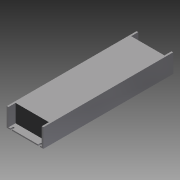
# Autodesk Inventor part: 5v_psu
Saved by Autodesk Inventor 2013 SP2 (Build 170200200, 200)
## iProperties
Created: 2018-10-22
Part Number: 5v_psu
Material: Generic
Document SubType Name: Modeling
Designer: alex
Density: 1 g/cm^3
Mass: 393.303 g
Surface Area: 466.03 cm^2
Volume: 393.303 cm^3
Author: alex
Autodesk Inventor part; units mm, degrees
ref_plane "YZ Plane" through (0, 0, 0) normal (1, 0, 0) x (0, 1, 0)
ref_plane "XZ Plane" through (0, 0, 0) normal (0, 1, 0) x (-1, 0, 0)
sketch "Sketch1" plane through (0, 0, 0) normal (0, 1, 0) x (-1, 0, 0)
  line L0 (34.1299, -113.6069) -> (-27.8701, -113.6069)
  line L1 (-27.8701, -113.6069) -> (-27.8701, 106.3931)
  line L2 (-27.8701, 106.3931) -> (34.1299, 106.3931)
  line L3 (34.1299, 106.3931) -> (34.1299, -113.6069)
  line L4 (34.1299, -113.6069) -> (-27.8701, 106.3931) construction
  line L5 (-27.8701, -113.6069) -> (34.1299, 106.3931) construction
  point P0 (0, 0)
  point P1 (3.1299, -3.6069)
  dimension "d0" = 62
  dimension "d1" = 220
  constraints: 12 end point, 2 midpoint, 2 parallel, 1 horizontal, 1 perpendicular
  measures "d0" distance of L1.end L2.end
  measures "d1" distance of L0.end L1.end
extrude "Extrusion1" add sketch "Sketch1" along normal blind 31.8
sketch "Sketch2" plane through (-34.1299, 0, 106.3931) normal (0, 0, 1) x (1, 0, 0)
  line L0 (62, 0) -> (0, 0) projected
  line L1 (62, 0) -> (62, 31.8) projected
  line L2 (0, 0) -> (0, 31.8) projected
  line L3 (2.8, 38.8076) -> (59.2, 38.8076)
  line L4 (59.2, 38.8076) -> (59.2, 2)
  line L5 (59.2, 2) -> (2.8, 2)
  line L6 (2.8, 2) -> (2.8, 38.8076)
  point P0 (34.1299, 0)
  dimension "d4" = 2.8
  dimension "d5" = 2.8
  dimension "d6" = 2
  constraints: 8 end point, 2 parallel, 1 horizontal, 1 perpendicular
  measures "d4" distance between parallel lines of L1 L4
  measures "d5" distance between parallel lines of L2 L6
  measures "d6" distance between parallel lines of L0 L5
extrude "Extrusion2" cut sketch "Sketch2" against normal blind 12
ref_plane "Work Plane1" through (27.8701, 0, -3.6069) normal (0, 0, -1) x (-1, 0, 0)
mirror "Mirror1" about plane through (27.8701, 0, -3.6069) normal (0, 0, -1) of "Extrusion2"
sketch "Sketch3" plane through (0, 0, 0) normal (0, -1, 0) x (1, 0, 0)
  line L0 (-34.1299, -113.6069) -> (27.8701, -113.6069) projected
  line L1 (27.8701, -113.6069) -> (27.8701, 106.3931) projected
  line L2 (27.8701, 106.3931) -> (-34.1299, 106.3931) projected
  line L3 (-34.1299, 106.3931) -> (-34.1299, -113.6069) projected
  line L4 (-26.6299, 106.3931) -> (-26.6299, 102.8931)
  circle A0 centre (-26.6299, 102.8931) radius 1.5
  line L5 (-28.1299, 102.8931) -> (-28.1299, 106.3931)
  line L6 (-25.1299, 102.8931) -> (-25.1299, 106.3931)
  line L7 (20.3701, 106.3931) -> (20.3701, 102.8931)
  circle A1 centre (20.3701, 102.8931) radius 1.5
  line L8 (21.8701, 102.8931) -> (21.8701, 106.3931)
  line L9 (18.8701, 102.8931) -> (18.8701, 106.3931)
  line L10 (-26.6299, -113.6069) -> (-26.6299, -110.1069)
  circle A2 centre (-26.6299, -110.1069) radius 1.5
  line L11 (-25.1299, -110.1069) -> (-25.1299, -113.6069)
  line L12 (-28.1299, -110.1069) -> (-28.1299, -113.6069)
  line L13 (20.3701, -113.6069) -> (20.3701, -110.1069)
  circle A3 centre (20.3701, -110.1069) radius 1.5
  line L14 (18.8701, -110.1069) -> (18.8701, -113.6069)
  line L15 (21.8701, -110.1069) -> (21.8701, -113.6069)
  point P0 (0, 0)
  dimension "d9" = 3
  dimension "d10" = 3.5
  dimension "d11" = 6
  dimension "d12" = 3.5
  dimension "d14" = 3
  dimension "d15" = 3.5
  dimension "d16" = 3
  dimension "d18" = 3.5
  dimension "d19" = 3
  dimension "d23" = 6
  dimension "d24" = 6
  dimension "d25" = 6
  constraints: 24 end point, 12 point on line, 9 perpendicular, 8 point on circle, 8 tangent, 4 centre point, 4 coincident, 3 parallel
  measures "d9" diameter of A0
  measures "d10" distance of L4.start L4.end
  measures "d11" distance between parallel lines of L3 L5
  measures "d12" distance of L7.start L7.end
  measures "d14" diameter of A1
  measures "d15" distance of L10.start L10.end
  measures "d16" diameter of A2
  measures "d18" distance of L13.start L13.end
  measures "d19" diameter of A3
  measures "d23" distance between parallel lines of L1 L8
  measures "d24" distance between parallel lines of L1 L15
  measures "d25" distance between parallel lines of L3 L12
extrude "Extrusion3" cut sketch "Sketch3" against normal blind 12 contours L12 A2 L10 L0 | L10 A2 L11 L0 | A2 | L2 L4 A0 L5 | L2 L6 A0 L4 | A0 | L14 A3 L13 L0 | L13 A3 L15 L0 | A3 | L2 L7 A1 L9 | L2 L8 A1 L7 | A1
body "Solid1"
